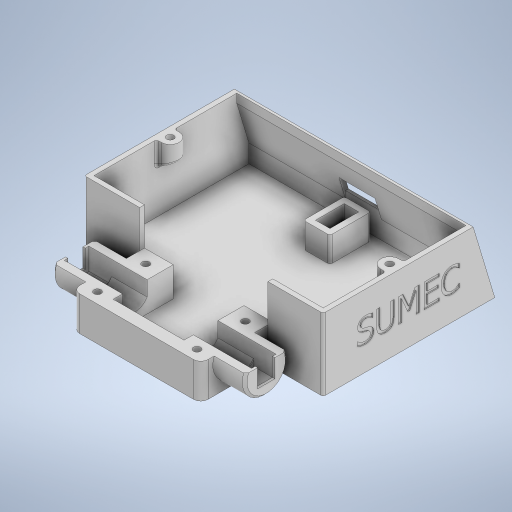
# Autodesk Inventor part: Tělo
Saved by Autodesk Inventor 2024 (Build 280153000, 153)
## iProperties
Created: 2023-04-15
Part Number: Tělo
Material: Všeobecné
Document SubType Name: Modeling
Designer: 42060
Density: 1 g/cm^3
Appearance: Výchozí
Author: 42060
Autodesk Inventor part; units mm, degrees
ref_plane "YZ Plane" through (0, 0, 0) normal (1, 0, 0) x (0, 1, 0)
ref_plane "XZ Plane" through (0, 0, 0) normal (0, 1, 0) x (-1, 0, 0)
ref_plane "XY Plane" through (0, 0, 0) normal (0, 0, 1) x (1, 0, 0)
sketch "Základ" plane through (0, 0, 0) normal (0, 0, 1) x (1, 0, 0)
  line L0 (0, 0) -> (49.75, 0)
  line L1 (49.75, 0) -> (49.75, -71.5)
  line L2 (49.75, -71.5) -> (26.75, -71.5)
  line L3 (26.75, -99.5) -> (0, -99.5)
  line L4 (0, -99.5) -> (0, 0)
  line L5 (0, -10) -> (47.75, -10)
  line L6 (47.75, -10) -> (47.75, -69.5)
  line L7 (47.75, -69.5) -> (14.75, -69.5)
  line L8 (14.75, -69.5) -> (14.75, -94.5)
  line L9 (14.75, -94.5) -> (0, -94.5)
  line L10 (26.75, -71.5) -> (26.75, -80.375)
  line L11 (26.75, -80.375) -> (26.75, -90.625)
  line L12 (26.75, -90.625) -> (26.75, -99.5)
  line L13 (26.75, -90.625) -> (14.75, -90.625)
  line L14 (26.75, -80.375) -> (14.75, -80.375)
  line L15 (26.75, -71.5) -> (26.75, -69.5)
  dimension "d0" = 49.75
  dimension "d1" = 99.5
  dimension "d3" = 2
  dimension "d5" = 28
  dimension "d14" = 10.25
  dimension "d15" = 12
  dimension "d16" = 5
  dimension "d17" = 23
  dimension "d18" = 2
  dimension "d19" = 10
  constraints: 32 end point, 8 perpendicular, 6 point on line, 3 horizontal, 2 collinear, 1 parallel, 1 vertical
  measures "d0" distance of L0.start L0.end
  measures "d1" distance between parallel lines of L3 L0
  measures "d3" distance between parallel lines of L1 L6
  measures "d5" distance of L2.end L3.start
  measures "d14" distance of L10.end L11.end
  measures "d15" distance between parallel lines of L8 L10
  measures "d16" distance between parallel lines of L9 L3
  measures "d17" distance between parallel lines of L1 L12
  measures "d18" distance between parallel lines of L2 L7
  measures "d19" distance between parallel lines of L0 L5
extrude "Podlaha" add sketch "Základ" along normal blind 2 contours L5 L6 L7 L8 L9 L4
extrude "Stěny" add sketch "Základ" along normal blind 30 contours L0 L1 L2 L15 L7 L6 L5 L4
extrude "Zadní stěny" add sketch "Základ" along normal blind 15 contours L9 L8 L13 L12 L3 L4 | L10 L14 L8 L7 L15
extrude "Stěna pod motorem" add sketch "Základ" along normal blind 5.25 contours L11 L13 L8 L14
sketch "Náčrt2" plane through (49.75, -71.5, 0) normal (1, 0, 0) x (0, 0, -1)
  line L0 (-2, 61.5) -> (-30, 61.5) projected
  line L1 (-2, 61.5) -> (-30, 61.5) projected
  line L2 (-30, 0) -> (-30, 71.5) projected
  line L3 (0, 71.5) -> (-30, 71.5) projected
  line L4 (0, 71.5) -> (0, 0) projected
  line L5 (-30, 62.5) -> (-10, 68.5)
  line L6 (-10, 68.5) -> (0, 71.5)
  dimension "d28" = 1
  dimension "d30" = 20
  constraints: 4 end point, 1 collinear, 1 point on line
  measures "d28" distance from line of L5.start L0
  measures "d30" horizontal distance of L5.end L5.start
extrude "Rampa" cut sketch "Náčrt2" against normal through all
sketch "Náčrt3" plane through (0, -10, 2) normal (-1, 0, 0) x (0, 0, 1)
  line L0 (0, 0) -> (28, 0) projected
  line L1 (0, 0) -> (28, 0) projected
  line L2 (24.3731, 0) -> (7.5, 5.0619)
  line L3 (7.5, 5.0619) -> (0, 5.0619)
  line L4 (0, 5.0619) -> (0, 0)
  line L5 (28, 1) -> (-2, 10) projected
  point P0 (-2, 10)
  point P1 (2, 7)
  point P2 (24.3731, 0)
  dimension "d34" = 7.5
  dimension "d37" = 2
  constraints: 6 end point, 1 horizontal, 1 perpendicular, 1 point on line, 2 other
  measures "d34" distance of L2.end L3.end
extrude "Přední rampa" cut sketch "Náčrt3" against normal up to surface (47.75 mm away)
sketch "Držák motoru" plane through (14.75, -94.5, 2) normal (-1, 0, 0) x (0, 0, 1)
  line L0 (3.25, 14.125) -> (13, 14.125) projected
  line L1 (3.25, 14.125) -> (3.25, 3.875) projected
  line L2 (3.25, 3.875) -> (13, 3.875) projected
  line L3 (6.13, 14.125) -> (12.37, 14.125)
  line L4 (12.37, 3.875) -> (6.13, 3.875)
  line L5 (3.25, 3.875) -> (13, 3.875) projected
  arc A0 (12.37, 3.875) -> (12.37, 14.125) centre (9.25, 9) ccw
  arc A1 (6.13, 14.125) -> (6.13, 3.875) centre (9.25, 9) ccw
  line L6 (15.25, 14.125) -> (15.25, 3.875) construction
  circle A2 centre (9.25, 9) radius 9
  line L7 (9.25, 18) -> (0, 18)
  line L8 (0, 0) -> (0, 89.5619) projected
  line L9 (0, 0) -> (13, 0) projected
  line L10 (13, -5) -> (13, 3.875) projected
  line L11 (0, 0) -> (13, 0) projected
  line L12 (0, 0) -> (13, 0) projected
  line L13 (12.37, 14.125) -> (12.37, 17.4419)
  line L14 (12.37, 3.875) -> (12.37, 0.5581)
  line L15 (12.37, 0.5581) -> (12.37, 0)
  line L16 (12.37, 17.4419) -> (12.37, 18)
  line L17 (12.37, 18) -> (9.25, 18)
  point P0 (-2, 94.5)
  point P1 (15.25, 9)
  point P2 (15.25, 9)
  point P3 (3.25, 9)
  point P4 (3.25, 9)
  point P5 (6.13, 3.875)
  point P6 (9.25, 0)
  point P7 (16.7333, 14)
  point P8 (16.7333, 4)
  point P9 (12.37, 0)
  dimension "d38" = 6
  dimension "d39" = 6
  dimension "d41" = 3
  dimension "d48" = 12
  constraints: 18 end point, 9 point on circle, 7 point on line, 4 tangent, 3 centre point, 3 coincident, 3 vertical, 2 horizontal alignment, 2 midpoint, 1 horizontal, 1 perpendicular
  measures "d38" radius of A0
  measures "d39" radius of A1
  measures "d41" radial gap between concentric circles of A2 A0
  measures "d48" distance between parallel lines of L1 L6
sketch "Náčrt10" plane through (14.75, -99.5, 0) normal (1, 0, 0) x (0, 0, -1)
  line L0 (-5.25, 8.875) -> (-15, 8.875) construction
  line L1 (-5.25, 8.875) -> (-17.25, 8.875) construction
  line L2 (-17.25, 8.875) -> (-17.25, 19.125) construction
  line L3 (-17.25, 19.125) -> (-5.25, 19.125) construction
  line L4 (-5.25, 19.125) -> (-5.25, 8.875) construction
  line L5 (-14.37, 8.875) -> (-8.13, 8.875)
  arc A0 (-8.13, 8.875) -> (-8.13, 19.125) centre (-11.25, 14) ccw
  line L6 (-14.37, 19.125) -> (-8.13, 19.125)
  arc A1 (-14.37, 5.5581) -> (-14.37, 22.4419) centre (-11.25, 14) ccw
  line L7 (-14.37, 8.875) -> (-14.37, 5.5581)
  line L8 (-14.37, 19.125) -> (-14.37, 22.4419)
  point P0 (0, 99.5)
  point P1 (-11.25, 19.125)
  point P2 (-11.25, 19.125)
  point P3 (-11.25, 8.875)
  point P4 (-11.25, 8.875)
  dimension "d79" = 12
  dimension "d80" = 6
  dimension "d81" = 18
  constraints: 16 end point, 5 point on line, 4 midpoint, 4 point on circle, 3 coincident, 2 centre point, 2 parallel, 2 perpendicular, 2 vertical alignment, 1 collinear, 1 horizontal, 1 horizontal alignment, 1 tangent
  measures "d79" distance between parallel lines of L4 L2
  measures "d80" radius of A0
  measures "d81" diameter of A1
extrude "Držák motoru (kulaté)" add sketch "Náčrt10" along normal blind 15
sketch "Náčrt11" plane through (29.75, -99.5, 0) normal (1, 0, 0) x (0, 0, -1)
  arc A0 (-8.13, 8.875) -> (-8.13, 19.125) centre (-11.25, 14) ccw projected
  circle A1 centre (-11.25, 14) radius 9
  line L0 (-17.25, 8.875) -> (-5.25, 8.875)
  line L1 (-5.25, 8.875) -> (-5.25, 19.125)
  line L2 (-5.25, 19.125) -> (-17.25, 19.125)
  line L3 (-17.25, 19.125) -> (-17.25, 8.875)
  line L4 (-17.25, 8.875) -> (-5.25, 19.125) construction
  line L5 (-5.25, 8.875) -> (-17.25, 19.125) construction
  line L6 (-14.37, 8.875) -> (-14.37, 5.5581) projected
  line L7 (-14.37, 22.4419) -> (-14.37, 19.125) projected
  point P0 (0, 99.5)
  dimension "d84" = 18
  constraints: 12 end point, 2 midpoint, 2 parallel, 1 centre point, 1 coincident, 1 horizontal, 1 horizontal alignment, 1 perpendicular, 1 tangent
  measures "d84" diameter of A1
extrude "Držák motoru (hranaté)" add sketch "Náčrt11" along normal blind 9.25 contours L0 L1 L2 L7 A1 L6
sketch "Spodní senzory" plane through (0, 0, 2) normal (0, 0, 1) x (1, 0, 0)
  line L0 (0, -4.9381) -> (47.75, -4.9381) projected
  line L1 (0, -94.5) -> (0, -4.9381) projected
  line L2 (0, -94.5) -> (14.75, -94.5) projected
  line L3 (14.75, -94.5) -> (14.75, -69.5) projected
  line L4 (14.75, -69.5) -> (47.75, -69.5) projected
  line L5 (47.75, -69.5) -> (47.75, -4.9381) projected
  line L6 (0, -24.4381) -> (5.5, -24.4381)
  line L7 (0, -21.9381) -> (3, -21.9381)
  line L8 (3, -21.9381) -> (3, -9.9381)
  line L9 (3, -9.9381) -> (0, -9.9381)
  line L10 (0, -7.4381) -> (5.5, -7.4381)
  line L11 (5.5, -7.4381) -> (5.5, -24.4381)
  point P0 (0, 0)
  dimension "d155" = 3
  dimension "d157" = 12
  dimension "d159" = 2.5
  dimension "d163" = 5
  dimension "d170" = 2.5
  dimension "d171" = 2.5
  constraints: 12 end point, 4 point on line, 3 horizontal, 2 perpendicular, 1 vertical
  measures "d155" distance of L7.start L7.end
  measures "d157" distance of L7.end L8.end
  measures "d159" distance between parallel lines of L7 L6
  measures "d163" distance between parallel lines of L0 L9
  measures "d170" distance between parallel lines of L10 L9
  measures "d171" distance between parallel lines of L8 L11
extrude "Spodní senzory (díra)" cut sketch "Spodní senzory" against normal through all contours L9 L8 L7 L1
extrude "Spodní senzory zvýšení" add sketch "Spodní senzory" along normal blind 10.5 contours L10 L11 L6 L1 L7 L8 L9
sketch "Náčrt12" plane through (0, 0, 15) normal (0, 0, 1) x (1, 0, 0)
  line L0 (26.75, -80.375) -> (26.75, -71.5) projected
  line L1 (26.75, -69.5) -> (26.75, -71.5) projected
  line L2 (26.75, -69.5) -> (14.75, -69.5) projected
  line L3 (14.75, -69.5) -> (14.75, -80.375) projected
  line L4 (14.75, -80.375) -> (26.75, -80.375) projected
  line L5 (26.75, -99.5) -> (26.75, -90.625) projected
  line L6 (26.75, -90.625) -> (14.75, -90.625) projected
  line L7 (14.75, -90.625) -> (14.75, -94.5) projected
  line L8 (14.75, -94.5) -> (0, -94.5) projected
  line L9 (0, -94.5) -> (0, -99.5) projected
  line L10 (0, -99.5) -> (26.75, -99.5) projected
  point P0 (0, 0)
extrude "Vyrovnání držáku motoru" cut sketch "Náčrt12" against normal up to surface (0.63 mm away)
sketch "Náčrt13" plane through (14.75, -80.375, 14.37) normal (0, 0, 1) x (1, 0, 0)
  line L0 (0, 0) -> (0, 10.875) projected
  line L1 (0, 10.875) -> (12, 10.875) projected
  line L2 (0, -14.125) -> (0, -10.25) projected
  line L3 (0, -10.25) -> (24.25, -10.25) projected
  point P0 (-14.75, 80.375)
  point P1 (6, 5.4375)
  point P2 (6, -14.6875)
  dimension "d89" = 6
  dimension "d90" = 5.4375
  dimension "d91" = 6
  dimension "d92" = 4.4375
  measures "d89" distance from line of L0 point (6, 5.438)
  measures "d90" distance from line of L1 point (6, 5.438)
  measures "d91" distance from line of L2 point (6, -14.687)
  measures "d92" distance from line of L3 point (6, -14.687)
hole "Díry pro objímku motoru" at (20.75, -95.0625, 14.37) at (20.75, -74.9375, 14.37) direction (0, 0, -1) diameter 3 depth 6
fillet "Zaoblení1" radius 3 1 edges at (26.75, -99.5, 7.185)
fillet "Zaoblení2" radius 1 1 edges at (49.75, -71.5, 15)
sketch "Náčrt14" plane through (39, -99.5, 0) normal (1, 0, 0) x (0, 0, -1)
  line L0 (-14.37, 19.125) -> (-5.25, 19.125) projected
  line L1 (-5.25, 19.125) -> (-5.25, 8.875) projected
  line L2 (-5.25, 8.875) -> (-14.37, 8.875) projected
  line L3 (-14.37, 8.875) -> (-14.37, 5.5581) projected
  arc A0 (-14.37, 5.5581) -> (-14.37, 22.4419) centre (-11.25, 14) ccw projected
  line L4 (-14.37, 22.4419) -> (-14.37, 19.125) projected
  line L5 (-14.37, 10.375) -> (-6.75, 10.375)
  line L6 (-6.75, 10.375) -> (-6.75, 17.625)
  line L7 (-6.75, 17.625) -> (-14.37, 17.625)
  line L8 (-14.37, 8.875) -> (-14.37, 10.375)
  line L9 (-14.37, 17.625) -> (-14.37, 19.125)
  point P0 (0, 99.5)
  dimension "d108" = 1.5
  dimension "d109" = 1.5
  dimension "d110" = 1.5
  constraints: 10 end point, 2 perpendicular, 2 point on line, 2 vertical, 2 vertical alignment
  measures "d108" distance between parallel lines of L5 L2
  measures "d109" distance between parallel lines of L1 L6
  measures "d110" distance between parallel lines of L0 L7
extrude "Vysunutí19" add sketch "Náčrt14" along normal blind 1
chamfer "Zkosení1" distance 1 angle 45 1 edges at (40, -85.5, 2.25)
chamfer "Zkosení2" distance 0.25 angle 45 2 edges at (29.75, -88.4394, 6.0193) (29.75, -82.5606, 6.0193)
sketch "Náčrt16" plane through (0, 0, 30) normal (0, 0, 1) x (1, 0, 0)
  line L0 (47.75, -36) -> (45.75, -36)
  arc A0 (45.75, -36) -> (45.75, -43.5) centre (45.75, -39.75) ccw
  line L1 (45.75, -43.5) -> (47.75, -43.5)
  line L2 (47.75, -10) -> (47.75, -69.5) projected
  point P0 (47.75, -39.75)
  point P1 (47.75, -39.75)
  point P2 (47.75, -39.75)
  dimension "d130" = 3.75
  dimension "d131" = 2
  constraints: 4 end point, 3 midpoint, 2 coincident, 2 point on circle, 2 point on line, 2 tangent, 1 centre point, 1 horizontal, 1 horizontal alignment, 1 parallel
  measures "d130" radius of A0
  measures "d131" distance of L1.start L1.end
extrude "Vysunutí20" add sketch "Náčrt16" against normal blind 10
sketch "Náčrt17" plane through (0, 0, 30) normal (0, 0, 1) x (1, 0, 0)
  arc A0 (45.75, -36) -> (45.75, -43.5) centre (45.75, -39.75) ccw projected
  point P0 (0, 0)
  constraints: 1 coincident
hole "Díra2" at (45.75, -39.75, 30) direction (0, 0, -1) diameter 3 depth 6
sketch "Náčrt18" plane through (45.75, -43.5, 30) normal (0, -1, 0) x (1, 0, 0)
  line L0 (-10.625, -22) -> (-25.625, -22) projected
  line L1 (-3.75, -10) -> (0, -10) projected
  line L2 (0, -10) -> (2, -10) projected
  line L3 (-3.75, 0) -> (-3.75, -10) projected
  line L4 (-3.75, -6.6802) -> (2, -10)
  point P0 (-45.75, -30)
  dimension "d141" = 30
  constraints: 2 end point, 1 point on line
  measures "d141" angle of L1 L4
extrude "Vysunutí21" cut sketch "Náčrt18" against normal blind 10
fillet "Zaoblení3" radius 1 9 edges at (46.75, -43.5, 20.5774) (46.75, -36, 20.5774) (43.0983, -42.4017, 22.6856) (43.0983, -37.0983, 22.6856) (47.75, -43.5, 25) (47.75, -36, 25) (47.75, -39.75, 20) (5.5, -24.4381, 7.25) (5.5, -7.4381, 7.25)
sketch "Náčrt20" plane through (0, -24.4381, 2) normal (0, -1, 0) x (1, 0, 0)
  line L0 (3, 10.5) -> (0, 10.5) projected
  line L1 (0, 10.5) -> (7.5, 10.5)
  line L2 (7.5, 10.5) -> (7.5, 16.5)
  line L3 (7.5, 16.5) -> (0, 16.5)
  line L4 (0, 16.5) -> (0, 10.5)
  point P0 (0, -2)
  dimension "d168" = 7.5
  dimension "d169" = 6
  constraints: 8 end point, 2 parallel, 1 horizontal, 1 perpendicular
  measures "d168" distance of L2.end L3.end
  measures "d169" distance of L1.end L2.end
extrude "Vysunutí22" cut sketch "Náčrt20" against normal through all
sketch "Náčrt21" plane through (0, 0, 2) normal (0, 0, 1) x (1, 0, 0)
  line L0 (0, -4.9381) -> (47.75, -4.9381) projected
  line L1 (0, -4.9381) -> (47.75, -4.9381) projected
  line L2 (7.5, -7.6381) -> (7.5, -5.8381) projected
  line L3 (7.5, -7.6381) -> (7.5, -5.55) projected
  line L4 (7.5, -3.75) -> (7.5, -5.55) projected
  line L5 (7.5, -5.8381) -> (7.5, -3.75) projected
  line L6 (0, -7.4381) -> (4.5, -7.4381) projected
  line L7 (4.5, -7.4381) -> (0, -7.4381) projected
  line L8 (7.5, -4.9381) -> (0, -4.9381)
  line L9 (0, -4.9381) -> (0, -7.4381)
  line L10 (0, -7.4381) -> (7.5, -7.4381)
  line L11 (7.5, -7.4381) -> (7.5, -4.9381)
  point P0 (0, 0)
  point P1 (7.5, -7.4381)
  point P2 (7.5, -4.9381)
  constraints: 8 end point, 2 parallel, 2 point on line, 1 horizontal, 1 perpendicular
extrude "Vysunutí23" cut sketch "Náčrt21" along normal up to surface (16.5 mm away)
mirror "Zrcadlení těla" about plane through (0, 0, 0) normal (1, 0, 0)
sketch "Náčrt15" plane through (49.75, -70.5, 0) normal (1, 0, 0) x (0, 0, -1)
  line L0 (-20.5, 12.75) -> (-20.5, 57.75) construction
  line L1 (-20.5, 57.75) -> (-9.5, 57.75) construction
  line L2 (-9.5, 57.75) -> (-9.5, 12.75) construction
  line L3 (-9.5, 12.75) -> (-20.5, 12.75) construction
  line L4 (-30, -1) -> (0, -1) projected
  line L5 (0, 0) -> (0, 70.5) projected
  spline S0 degree 2 poles (-10.1434, 16.5506) (-10.1434, 15.4647) (-10.5972, 13.9412) (-10.9214, 13.2686) knots 0 0 0 1 2 2 2
  line L6 (-10.9214, 13.2686) -> (-12.5908, 13.2686)
  line L7 (-12.5908, 13.2686) -> (-12.5908, 13.3659)
  spline S1 degree 2 poles (-12.5908, 13.3659) (-11.9749, 14.0223) (-11.2942, 15.6835) (-11.2942, 16.4534) knots 0 0 0 1 2 2 2
  spline S2 degree 2 poles (-11.2942, 16.4534) (-11.2942, 17.5555) (-12.2099, 18.6819) (-12.9635, 18.6819) knots 0 0 0 1 2 2 2
  spline S3 degree 2 poles (-12.9635, 18.6819) (-13.5632, 18.6819) (-14.3088, 18.0904) (-14.4951, 17.4502) knots 0 0 0 1 2 2 2
  spline S4 degree 2 poles (-14.4951, 17.4502) (-14.6248, 16.9882) (-14.8031, 16.2184) (-14.9489, 15.643) knots 0 0 0 1 2 2 2
  spline S5 degree 2 poles (-14.9489, 15.643) (-15.0867, 15.1244) (-15.5, 14.3059) (-15.8323, 13.9899) knots 0 0 0 1 2 2 2
  spline S6 degree 2 poles (-15.8323, 13.9899) (-16.1645, 13.6819) (-17.0559, 13.3416) (-17.6394, 13.3416) knots 0 0 0 1 2 2 2
  spline S7 degree 2 poles (-17.6394, 13.3416) (-18.8549, 13.3416) (-20.5, 15.2378) (-20.5, 16.7046) knots 0 0 0 1 2 2 2
  spline S8 degree 2 poles (-20.5, 16.7046) (-20.5, 17.5474) (-20.1677, 19.0385) (-19.8517, 19.6787) knots 0 0 0 1 2 2 2
  line L8 (-19.8517, 19.6787) -> (-18.2634, 19.6787)
  line L9 (-18.2634, 19.6787) -> (-18.2634, 19.5814)
  spline S9 degree 2 poles (-18.2634, 19.5814) (-18.701, 19.1033) (-19.3493, 17.6122) (-19.3493, 16.7938) knots 0 0 0 1 2 2 2
  spline S10 degree 2 poles (-19.3493, 16.7938) (-19.3493, 15.8699) (-18.4822, 14.7273) (-17.7771, 14.7273) knots 0 0 0 1 2 2 2
  spline S11 degree 2 poles (-17.7771, 14.7273) (-17.1451, 14.7273) (-16.3914, 15.3999) (-16.2212, 16.032) knots 0 0 0 1 2 2 2
  spline S12 degree 2 poles (-16.2212, 16.032) (-16.1078, 16.4534) (-15.816, 17.6771) (-15.6945, 18.0823) knots 0 0 0 1 2 2 2
  spline S13 degree 2 poles (-15.6945, 18.0823) (-15.3784, 19.1114) (-14.1062, 20.0677) (-13.1742, 20.0677) knots 0 0 0 1 2 2 2
  spline S14 degree 2 poles (-13.1742, 20.0677) (-12.5827, 20.0677) (-11.4481, 19.5895) (-11.0511, 19.16) knots 0 0 0 1 2 2 2
  spline S15 degree 2 poles (-11.0511, 19.16) (-10.6135, 18.6819) (-10.1434, 17.4664) (-10.1434, 16.5506) knots 0 0 0 1 2 2 2
  spline S16 degree 2 poles (-10.111, 24.9137) (-10.111, 24.0304) (-10.5729, 22.7176) (-11.0348, 22.2557) knots 0 0 0 1 2 2 2
  spline S17 degree 2 poles (-11.0348, 22.2557) (-11.5535, 21.7289) (-13.0122, 21.2994) (-14.0818, 21.2994) knots 0 0 0 1 2 2 2
  line L10 (-14.0818, 21.2994) -> (-20.3217, 21.2994)
  line L11 (-20.3217, 21.2994) -> (-20.3217, 22.6284)
  line L12 (-20.3217, 22.6284) -> (-14.0818, 22.6284)
  spline S18 degree 2 poles (-14.0818, 22.6284) (-13.3849, 22.6284) (-12.4449, 22.8067) (-12.064, 23.0579) knots 0 0 0 1 2 2 2
  spline S19 degree 2 poles (-12.064, 23.0579) (-11.6588, 23.3254) (-11.2455, 24.2492) (-11.2455, 24.9137) knots 0 0 0 1 2 2 2
  spline S20 degree 2 poles (-11.2455, 24.9137) (-11.2455, 25.5377) (-11.6588, 26.5101) (-12.064, 26.7776) knots 0 0 0 1 2 2 2
  spline S21 degree 2 poles (-12.064, 26.7776) (-12.4449, 27.0288) (-13.3768, 27.2071) (-14.0494, 27.2071) knots 0 0 0 1 2 2 2
  line L13 (-14.0494, 27.2071) -> (-20.3217, 27.2071)
  line L14 (-20.3217, 27.2071) -> (-20.3217, 28.5361)
  line L15 (-20.3217, 28.5361) -> (-14.0818, 28.5361)
  spline S22 degree 2 poles (-14.0818, 28.5361) (-13.0365, 28.5361) (-11.5454, 28.1147) (-11.0348, 27.5798) knots 0 0 0 1 2 2 2
  spline S23 degree 2 poles (-11.0348, 27.5798) (-10.5648, 27.1017) (-10.111, 25.8375) (-10.111, 24.9137) knots 0 0 0 1 2 2 2
  line L16 (-10.3217, 39.0142) -> (-10.3217, 37.6852)
  line L17 (-10.3217, 37.6852) -> (-18.936, 37.6852)
  line L18 (-18.936, 37.6852) -> (-13.077, 35.0758)
  line L19 (-13.077, 35.0758) -> (-13.077, 34.2654)
  line L20 (-13.077, 34.2654) -> (-18.936, 31.6803)
  line L21 (-18.936, 31.6803) -> (-10.3217, 31.6803)
  line L22 (-10.3217, 31.6803) -> (-10.3217, 30.4404)
  line L23 (-10.3217, 30.4404) -> (-20.3217, 30.4404)
  line L24 (-20.3217, 30.4404) -> (-20.3217, 32.2557)
  line L25 (-20.3217, 32.2557) -> (-14.7545, 34.7516)
  line L26 (-14.7545, 34.7516) -> (-20.3217, 37.1665)
  line L27 (-20.3217, 37.1665) -> (-20.3217, 39.0142)
  line L28 (-20.3217, 39.0142) -> (-10.3217, 39.0142)
  line L29 (-10.3217, 41.0401) -> (-20.3217, 41.0401)
  line L30 (-20.3217, 41.0401) -> (-20.3217, 47.2962)
  line L31 (-20.3217, 47.2962) -> (-19.1386, 47.2962)
  line L32 (-19.1386, 47.2962) -> (-19.1386, 42.3691)
  line L33 (-19.1386, 42.3691) -> (-16.3995, 42.3691)
  line L34 (-16.3995, 42.3691) -> (-16.3995, 46.9639)
  line L35 (-16.3995, 46.9639) -> (-15.2164, 46.9639)
  line L36 (-15.2164, 46.9639) -> (-15.2164, 42.3691)
  line L37 (-15.2164, 42.3691) -> (-11.5049, 42.3691)
  line L38 (-11.5049, 42.3691) -> (-11.5049, 47.2962)
  line L39 (-11.5049, 47.2962) -> (-10.3217, 47.2962)
  line L40 (-10.3217, 47.2962) -> (-10.3217, 41.0401)
  spline S24 degree 2 poles (-10.1434, 52.6609) (-10.1434, 51.6884) (-10.7998, 50.0434) (-11.4562, 49.4437) knots 0 0 0 1 2 2 2
  spline S25 degree 2 poles (-11.4562, 49.4437) (-12.1045, 48.844) (-14.0494, 48.1876) (-15.3136, 48.1876) knots 0 0 0 1 2 2 2
  spline S26 degree 2 poles (-15.3136, 48.1876) (-16.5697, 48.1876) (-18.4335, 48.8278) (-19.1224, 49.4356) knots 0 0 0 1 2 2 2
  spline S27 degree 2 poles (-19.1224, 49.4356) (-19.795, 50.0353) (-20.5, 51.6722) (-20.5, 52.6852) knots 0 0 0 1 2 2 2
  spline S28 degree 2 poles (-20.5, 52.6852) (-20.5, 53.1876) (-20.3541, 54.0709) (-20.2407, 54.4437) knots 0 0 0 1 2 2 2
  spline S29 degree 2 poles (-20.2407, 54.4437) (-20.1353, 54.7678) (-19.8355, 55.4404) (-19.6572, 55.7727) knots 0 0 0 1 2 2 2
  line L41 (-19.6572, 55.7727) -> (-18.0527, 55.7727)
  line L42 (-18.0527, 55.7727) -> (-18.0527, 55.6673)
  spline S30 degree 2 poles (-18.0527, 55.6673) (-18.2147, 55.4891) (-18.6686, 54.938) (-18.8874, 54.5409) knots 0 0 0 1 2 2 2
  spline S31 degree 2 poles (-18.8874, 54.5409) (-19.0981, 54.16) (-19.3655, 53.2605) (-19.3655, 52.6771) knots 0 0 0 1 2 2 2
  spline S32 degree 2 poles (-19.3655, 52.6771) (-19.3655, 52.0369) (-18.8387, 50.8942) (-18.3363, 50.4647) knots 0 0 0 1 2 2 2
  spline S33 degree 2 poles (-18.3363, 50.4647) (-17.8258, 50.0434) (-16.278, 49.5733) (-15.3136, 49.5733) knots 0 0 0 1 2 2 2
  spline S34 degree 2 poles (-15.3136, 49.5733) (-14.2844, 49.5733) (-12.8015, 50.0677) (-12.2909, 50.4972) knots 0 0 0 1 2 2 2
  spline S35 degree 2 poles (-12.2909, 50.4972) (-11.7966, 50.9186) (-11.2942, 52.045) (-11.2942, 52.6771) knots 0 0 0 1 2 2 2
  spline S36 degree 2 poles (-11.2942, 52.6771) (-11.2942, 53.2524) (-11.5778, 54.233) (-11.7885, 54.6139) knots 0 0 0 1 2 2 2
  spline S37 degree 2 poles (-11.7885, 54.6139) (-11.9992, 54.9785) (-12.4368, 55.5215) (-12.5908, 55.6754) knots 0 0 0 1 2 2 2
  line L43 (-12.5908, 55.6754) -> (-12.5908, 55.7727)
  line L44 (-12.5908, 55.7727) -> (-11.0024, 55.7727)
  spline S38 degree 2 poles (-11.0024, 55.7727) (-10.8485, 55.4404) (-10.5648, 54.857) (-10.4352, 54.4437) knots 0 0 0 1 2 2 2
  spline S39 degree 2 poles (-10.4352, 54.4437) (-10.2893, 54.0061) (-10.1434, 53.2605) (-10.1434, 52.6609) knots 0 0 0 1 2 2 2
  point P0 (-15, 12.75)
  point P1 (-15, -1)
  point P2 (-9.5, 35.25)
  point P3 (0, 35.25)
  dimension "d145" = 11
  dimension "d146" = 45
  constraints: 4 midpoint, 1 horizontal alignment, 1 vertical alignment, 2 other
  measures "d145" distance of L0.end L1.end
  measures "d146" distance of L1.end L2.end
emboss "Reliéf1" sketch "Náčrt15" operation cut depth 0.4 direction (-1, 0, 0)
sketch "Náčrt19" plane through (-49.75, -70.5, 0) normal (-1, 0, 0) x (0, 0, 1)
  line L0 (20.5, 57.75) -> (20.5, 12.75) construction
  line L1 (20.5, 12.75) -> (9.5, 12.75) construction
  line L2 (9.5, 12.75) -> (9.5, 57.75) construction
  line L3 (9.5, 57.75) -> (20.5, 57.75) construction
  line L4 (30, -1) -> (0, -1) projected
  line L5 (0, 0) -> (0, 70.5) projected
  spline S0 degree 2 poles (10.1434, 53.9494) (10.1434, 55.0353) (10.5972, 56.5588) (10.9214, 57.2314) knots 0 0 0 1 2 2 2
  line L6 (10.9214, 57.2314) -> (12.5908, 57.2314)
  line L7 (12.5908, 57.2314) -> (12.5908, 57.1341)
  spline S1 degree 2 poles (12.5908, 57.1341) (11.9749, 56.4777) (11.2942, 54.8165) (11.2942, 54.0466) knots 0 0 0 1 2 2 2
  spline S2 degree 2 poles (11.2942, 54.0466) (11.2942, 52.9445) (12.2099, 51.8181) (12.9635, 51.8181) knots 0 0 0 1 2 2 2
  spline S3 degree 2 poles (12.9635, 51.8181) (13.5632, 51.8181) (14.3088, 52.4096) (14.4951, 53.0498) knots 0 0 0 1 2 2 2
  spline S4 degree 2 poles (14.4951, 53.0498) (14.6248, 53.5118) (14.8031, 54.2816) (14.9489, 54.857) knots 0 0 0 1 2 2 2
  spline S5 degree 2 poles (14.9489, 54.857) (15.0867, 55.3756) (15.5, 56.1941) (15.8323, 56.5101) knots 0 0 0 1 2 2 2
  spline S6 degree 2 poles (15.8323, 56.5101) (16.1645, 56.8181) (17.0559, 57.1584) (17.6394, 57.1584) knots 0 0 0 1 2 2 2
  spline S7 degree 2 poles (17.6394, 57.1584) (18.8549, 57.1584) (20.5, 55.2622) (20.5, 53.7954) knots 0 0 0 1 2 2 2
  spline S8 degree 2 poles (20.5, 53.7954) (20.5, 52.9526) (20.1677, 51.4615) (19.8517, 50.8213) knots 0 0 0 1 2 2 2
  line L8 (19.8517, 50.8213) -> (18.2634, 50.8213)
  line L9 (18.2634, 50.8213) -> (18.2634, 50.9186)
  spline S9 degree 2 poles (18.2634, 50.9186) (18.701, 51.3967) (19.3493, 52.8878) (19.3493, 53.7062) knots 0 0 0 1 2 2 2
  spline S10 degree 2 poles (19.3493, 53.7062) (19.3493, 54.6301) (18.4822, 55.7727) (17.7771, 55.7727) knots 0 0 0 1 2 2 2
  spline S11 degree 2 poles (17.7771, 55.7727) (17.1451, 55.7727) (16.3914, 55.1001) (16.2212, 54.468) knots 0 0 0 1 2 2 2
  spline S12 degree 2 poles (16.2212, 54.468) (16.1078, 54.0466) (15.816, 52.8229) (15.6945, 52.4177) knots 0 0 0 1 2 2 2
  spline S13 degree 2 poles (15.6945, 52.4177) (15.3784, 51.3886) (14.1062, 50.4323) (13.1742, 50.4323) knots 0 0 0 1 2 2 2
  spline S14 degree 2 poles (13.1742, 50.4323) (12.5827, 50.4323) (11.4481, 50.9105) (11.0511, 51.34) knots 0 0 0 1 2 2 2
  spline S15 degree 2 poles (11.0511, 51.34) (10.6135, 51.8181) (10.1434, 53.0336) (10.1434, 53.9494) knots 0 0 0 1 2 2 2
  spline S16 degree 2 poles (10.111, 45.5863) (10.111, 46.4696) (10.5729, 47.7824) (11.0348, 48.2443) knots 0 0 0 1 2 2 2
  spline S17 degree 2 poles (11.0348, 48.2443) (11.5535, 48.7711) (13.0122, 49.2006) (14.0818, 49.2006) knots 0 0 0 1 2 2 2
  line L10 (14.0818, 49.2006) -> (20.3217, 49.2006)
  line L11 (20.3217, 49.2006) -> (20.3217, 47.8716)
  line L12 (20.3217, 47.8716) -> (14.0818, 47.8716)
  spline S18 degree 2 poles (14.0818, 47.8716) (13.3849, 47.8716) (12.4449, 47.6933) (12.064, 47.4421) knots 0 0 0 1 2 2 2
  spline S19 degree 2 poles (12.064, 47.4421) (11.6588, 47.1746) (11.2455, 46.2508) (11.2455, 45.5863) knots 0 0 0 1 2 2 2
  spline S20 degree 2 poles (11.2455, 45.5863) (11.2455, 44.9623) (11.6588, 43.9899) (12.064, 43.7224) knots 0 0 0 1 2 2 2
  spline S21 degree 2 poles (12.064, 43.7224) (12.4449, 43.4712) (13.3768, 43.2929) (14.0494, 43.2929) knots 0 0 0 1 2 2 2
  line L13 (14.0494, 43.2929) -> (20.3217, 43.2929)
  line L14 (20.3217, 43.2929) -> (20.3217, 41.9639)
  line L15 (20.3217, 41.9639) -> (14.0818, 41.9639)
  spline S22 degree 2 poles (14.0818, 41.9639) (13.0365, 41.9639) (11.5454, 42.3853) (11.0348, 42.9202) knots 0 0 0 1 2 2 2
  spline S23 degree 2 poles (11.0348, 42.9202) (10.5648, 43.3983) (10.111, 44.6625) (10.111, 45.5863) knots 0 0 0 1 2 2 2
  line L16 (10.3217, 31.4858) -> (10.3217, 32.8148)
  line L17 (10.3217, 32.8148) -> (18.936, 32.8148)
  line L18 (18.936, 32.8148) -> (13.077, 35.4242)
  line L19 (13.077, 35.4242) -> (13.077, 36.2346)
  line L20 (13.077, 36.2346) -> (18.936, 38.8197)
  line L21 (18.936, 38.8197) -> (10.3217, 38.8197)
  line L22 (10.3217, 38.8197) -> (10.3217, 40.0596)
  line L23 (10.3217, 40.0596) -> (20.3217, 40.0596)
  line L24 (20.3217, 40.0596) -> (20.3217, 38.2443)
  line L25 (20.3217, 38.2443) -> (14.7545, 35.7484)
  line L26 (14.7545, 35.7484) -> (20.3217, 33.3335)
  line L27 (20.3217, 33.3335) -> (20.3217, 31.4858)
  line L28 (20.3217, 31.4858) -> (10.3217, 31.4858)
  line L29 (10.3217, 29.4599) -> (20.3217, 29.4599)
  line L30 (20.3217, 29.4599) -> (20.3217, 23.2038)
  line L31 (20.3217, 23.2038) -> (19.1386, 23.2038)
  line L32 (19.1386, 23.2038) -> (19.1386, 28.1309)
  line L33 (19.1386, 28.1309) -> (16.3995, 28.1309)
  line L34 (16.3995, 28.1309) -> (16.3995, 23.5361)
  line L35 (16.3995, 23.5361) -> (15.2164, 23.5361)
  line L36 (15.2164, 23.5361) -> (15.2164, 28.1309)
  line L37 (15.2164, 28.1309) -> (11.5049, 28.1309)
  line L38 (11.5049, 28.1309) -> (11.5049, 23.2038)
  line L39 (11.5049, 23.2038) -> (10.3217, 23.2038)
  line L40 (10.3217, 23.2038) -> (10.3217, 29.4599)
  spline S24 degree 2 poles (10.1434, 17.8391) (10.1434, 18.8116) (10.7998, 20.4566) (11.4562, 21.0563) knots 0 0 0 1 2 2 2
  spline S25 degree 2 poles (11.4562, 21.0563) (12.1045, 21.656) (14.0494, 22.3124) (15.3136, 22.3124) knots 0 0 0 1 2 2 2
  spline S26 degree 2 poles (15.3136, 22.3124) (16.5697, 22.3124) (18.4335, 21.6722) (19.1224, 21.0644) knots 0 0 0 1 2 2 2
  spline S27 degree 2 poles (19.1224, 21.0644) (19.795, 20.4647) (20.5, 18.8278) (20.5, 17.8148) knots 0 0 0 1 2 2 2
  spline S28 degree 2 poles (20.5, 17.8148) (20.5, 17.3124) (20.3541, 16.4291) (20.2407, 16.0563) knots 0 0 0 1 2 2 2
  spline S29 degree 2 poles (20.2407, 16.0563) (20.1353, 15.7322) (19.8355, 15.0596) (19.6572, 14.7273) knots 0 0 0 1 2 2 2
  line L41 (19.6572, 14.7273) -> (18.0527, 14.7273)
  line L42 (18.0527, 14.7273) -> (18.0527, 14.8327)
  spline S30 degree 2 poles (18.0527, 14.8327) (18.2147, 15.0109) (18.6686, 15.562) (18.8874, 15.9591) knots 0 0 0 1 2 2 2
  spline S31 degree 2 poles (18.8874, 15.9591) (19.0981, 16.34) (19.3655, 17.2395) (19.3655, 17.8229) knots 0 0 0 1 2 2 2
  spline S32 degree 2 poles (19.3655, 17.8229) (19.3655, 18.4631) (18.8387, 19.6058) (18.3363, 20.0353) knots 0 0 0 1 2 2 2
  spline S33 degree 2 poles (18.3363, 20.0353) (17.8258, 20.4566) (16.278, 20.9267) (15.3136, 20.9267) knots 0 0 0 1 2 2 2
  spline S34 degree 2 poles (15.3136, 20.9267) (14.2844, 20.9267) (12.8015, 20.4323) (12.2909, 20.0028) knots 0 0 0 1 2 2 2
  spline S35 degree 2 poles (12.2909, 20.0028) (11.7966, 19.5814) (11.2942, 18.455) (11.2942, 17.8229) knots 0 0 0 1 2 2 2
  spline S36 degree 2 poles (11.2942, 17.8229) (11.2942, 17.2476) (11.5778, 16.267) (11.7885, 15.8861) knots 0 0 0 1 2 2 2
  spline S37 degree 2 poles (11.7885, 15.8861) (11.9992, 15.5215) (12.4368, 14.9785) (12.5908, 14.8246) knots 0 0 0 1 2 2 2
  line L43 (12.5908, 14.8246) -> (12.5908, 14.7273)
  line L44 (12.5908, 14.7273) -> (11.0024, 14.7273)
  spline S38 degree 2 poles (11.0024, 14.7273) (10.8485, 15.0596) (10.5648, 15.643) (10.4352, 16.0563) knots 0 0 0 1 2 2 2
  spline S39 degree 2 poles (10.4352, 16.0563) (10.2893, 16.4939) (10.1434, 17.2395) (10.1434, 17.8391) knots 0 0 0 1 2 2 2
  point P0 (15, 12.75)
  point P1 (15, -1)
  point P2 (9.5, 35.25)
  point P3 (0, 35.25)
  dimension "d149" = 11
  dimension "d150" = 45
  constraints: 4 midpoint, 1 horizontal alignment, 1 vertical alignment, 2 other
  measures "d149" distance of L0.end L1.end
  measures "d150" distance of L1.end L2.end
emboss "Reliéf2" sketch "Náčrt19" operation cut depth 0.4 direction (1, 0, 0)
